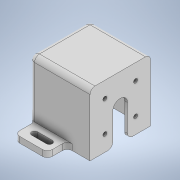
# Autodesk Inventor part: NEMA17_Shroud
Saved by Autodesk Inventor 2021 (Build 250183000, 183)
## iProperties
Created: 2021-10-06
Part Number: NEMA17_Shroud
Material: Generic
Document SubType Name: Modeling
Designer: Jorian Brusind
Density: 1 g/cm^3
Appearance: Default
Author: Jorian Brusind
Autodesk Inventor part; units mm, degrees
ref_plane "YZ Plane" through (0, 0, 0) normal (1, 0, 0) x (0, 1, 0)
sketch "Sketch1" plane through (0, 0, 0) normal (0, 1, 0) x (-1, 0, 0)
  line L0 (0, 0) -> (55, 0)
  line L1 (55, 0) -> (55, -55)
  line L2 (55, -55) -> (0, -55)
  line L3 (0, -58) -> (58, -58)
  line L4 (58, -58) -> (58, 3)
  line L5 (58, 3) -> (0, 3)
  line L6 (0, 3) -> (0, 0)
  line L7 (0, -55) -> (0, -58)
  dimension "d0" = 55
  dimension "d1" = 55
  dimension "d2" = 3
  constraints: 16 end point, 3 equal length, 2 perpendicular, 1 horizontal, 1 vertical, 2 other
  measures "d0" distance of L1.end L2.end
  measures "d1" distance of L0.end L1.end
  measures "d2" distance between parallel lines of L1 L4
extrude "Extrusion1" add sketch "Sketch1" along normal blind 60
sketch "Sketch2" plane through (0, 60, 0) normal (0, 1, 0) x (1, 0, 0)
  line L0 (-58, 58) -> (-58, -3) projected
  line L1 (0, 55) -> (0, 58) projected
  line L2 (-58, -3) -> (0, -3)
  line L3 (0, -3) -> (0, 58)
  line L4 (0, 58) -> (-58, 58)
  line L5 (-58, 58) -> (-58, -3)
  point P0 (0, 0)
  constraints: 8 end point, 2 parallel, 1 horizontal, 1 perpendicular
extrude "Extrusion2" add sketch "Sketch2" along normal blind 3
ref_plane "Work Plane1" through (0, -5, 0) normal (0, -1, 0) x (1, 0, 0)
ref_plane "Work Plane2" through (5, 60, 0) normal (1, 0, 0) x (0, 0, -1)
fillet "Fillet11" radius 5 3 edges at (-29, 63, 3) (-29, 63, -58) (-58, 63, -27.5)
fillet "Fillet12" radius 5 4 edges at (-56.5355, 61.5355, 1.5355) (-58, 29, 3) (-56.5355, 61.5355, -56.5355) (-58, 29, -58)
sketch "Sketch5" plane through (0, 0, 0) normal (0, -1, 0) x (1, 0, 0)
  line L0 (-53, -58) -> (-20, -58)
  line L1 (-20, -58) -> (-20, -78)
  line L2 (-20, -78) -> (-53, -78)
  line L3 (-53, -78) -> (-53, -58)
  line L4 (-58, -53) -> (-58, -2) projected
  line L5 (-53, -68) -> (-43, -68)
  line L6 (-43, -68) -> (-28, -68) construction
  line L7 (-43, -71) -> (-28, -71)
  line L8 (-28, -65) -> (-43, -65)
  arc A0 (-43, -65) -> (-43, -71) centre (-43, -68) ccw
  arc A1 (-28, -71) -> (-28, -65) centre (-28, -68) ccw
  line L9 (-53, 3) -> (0, 3) projected
  line L10 (-53, 3) -> (-20, 3)
  line L11 (-20, 3) -> (-20, 23)
  line L12 (-20, 23) -> (-53, 23)
  line L13 (-53, 23) -> (-53, 3)
  line L14 (-53, 13) -> (-43, 13)
  line L15 (-43, 13) -> (-28, 13) construction
  line L16 (-43, 10) -> (-28, 10)
  line L17 (-28, 16) -> (-43, 16)
  arc A2 (-43, 16) -> (-43, 10) centre (-43, 13) ccw
  arc A3 (-28, 10) -> (-28, 16) centre (-28, 13) ccw
  line L18 (-43, 13) -> (-28, 13) construction
  point P0 (-35.5, -68)
  point P1 (-35.5, 13)
  dimension "d70" = 33
  dimension "d71" = 20
  dimension "d72" = 5
  dimension "d74" = 10
  dimension "d75" = 15
  dimension "d76" = 6
  dimension "d77" = 33
  dimension "d78" = 20
  dimension "d79" = 10
  dimension "d80" = 15
  dimension "d81" = 0
  dimension "d82" = 6
  constraints: 38 end point, 8 point on circle, 8 tangent, 7 horizontal, 6 parallel, 4 centre point, 4 midpoint, 2 perpendicular, 1 collinear
  measures "d70" distance of L1.end L2.end
  measures "d71" distance of L0.end L1.end
  measures "d72" distance between parallel lines of L4 L3
  measures "d74" distance of L5.start L5.end
  measures "d75" distance of L5.end L6.end
  measures "d76" diameter of A1
  measures "d77" distance of L12.end L11.end
  measures "d78" distance of L11.end L10.end
  measures "d79" distance of L14.start L14.end
  measures "d80" distance of L14.end L15.end
  measures "d81" distance between parallel lines of L15 L18
  measures "d82" diameter of A3
extrude "Extrusion5" add sketch "Sketch5" against normal blind 6
sketch "Sketch6" plane through (0, 60, 0) normal (1, 0, 0) x (0, 0, -1)
  line L0 (58, -52) -> (58, -60) projected
  line L1 (-3, 3) -> (58, 3)
  line L2 (58, 3) -> (58, -60)
  line L3 (58, -60) -> (-3, -60)
  line L4 (-3, -60) -> (-3, 3)
  point P0 (0, -60)
  dimension "d52" = 61
  constraints: 8 end point, 2 parallel, 1 horizontal, 1 perpendicular
  measures "d52" distance between parallel lines of L2 L4
extrude "Extrusion6" add sketch "Sketch6" along normal blind 3
fillet "Fillet14" radius 5 2 edges at (1.5, 63, -58) (1.5, 63, 3)
sketch "Sketch7" plane through (3, 60, 0) normal (1, 0, 0) x (0, 0, -1)
  line L0 (58, 3) -> (-3, 3) projected
  line L1 (27.5, 3) -> (27.5, -13)
  line L2 (0, -60) -> (55, -60) projected
  line L3 (58, -60) -> (58, 3) projected
  line L4 (58, -13) -> (43, -13)
  line L5 (-3, 3) -> (-3, -60) projected
  circle A0 centre (43, -13) radius 2
  circle A1 centre (43, -44) radius 2
  circle A2 centre (12, -13) radius 2
  circle A3 centre (12, -44) radius 2
  point P0 (53, 3)
  point P1 (2, 3)
  point P2 (58, -2)
  point P3 (-3, -2)
  dimension "d56" = 16
  dimension "d57" = 15
  dimension "d58" = 4
  dimension "d61" = 31
  dimension "d64" = 31
  dimension "d67" = 16
  constraints: 4 centre point, 4 end point, 2 perpendicular, 1 coincident, 1 horizontal, 1 midpoint, 1 point on line, 1 vertical, 6 other
  measures "d56" distance of L1.start L1.end
  measures "d57" distance of L4.start L4.end
  measures "d58" diameter of A0
  measures "d61" distance of A0.centre A1.centre
  measures "d64" distance of A0.centre A2.centre
  measures "d67" distance from line of L0 L4.end
extrude "Extrusion7" cut sketch "Sketch7" against normal up to surface (3 mm away)
fillet "Fillet15" radius 5 8 edges at (-20, 3, 23) (-20, 3, 3) (-20, 3, -78) (-53, 3, 23) (-53, 3, 3) (-53, 3, -78) (-53, 3, -58) (-20, 3, -58)
sketch "Sketch8" plane through (3, 60, 0) normal (1, 0, 0) x (0, 0, -1)
  line L0 (58, -2) -> (58, -54) projected
  line L1 (58, -28) -> (27.5, -28)
  circle A0 centre (27.5, -28) radius 7.5
  line L2 (27.5, -28) -> (20, -28)
  line L3 (27.5, -28) -> (35, -28)
  line L4 (35, -28) -> (35, -60)
  line L5 (53, -60) -> (2, -60) projected
  line L6 (20, -28) -> (20, -60)
  line L7 (20, -60) -> (35, -60)
  point P0 (0, -60)
  dimension "d84" = 30.5
  dimension "d85" = 15
  dimension "d86" = 32
  dimension "d87" = 32
  constraints: 12 end point, 3 point on line, 2 horizontal, 2 point on circle, 1 centre point, 1 coincident, 1 collinear, 1 midpoint
  measures "d84" distance of L1.start L1.end
  measures "d85" diameter of A0
  measures "d86" distance of L3.end L4.end
  measures "d87" distance of L2.end L6.end
extrude "Extrusion8" cut sketch "Sketch8" against normal up to surface (3 mm away)
fillet "Fillet16" radius 5 2 edges at (1.5, 0, -35) (1.5, 0, -20)
body "Solid1"
